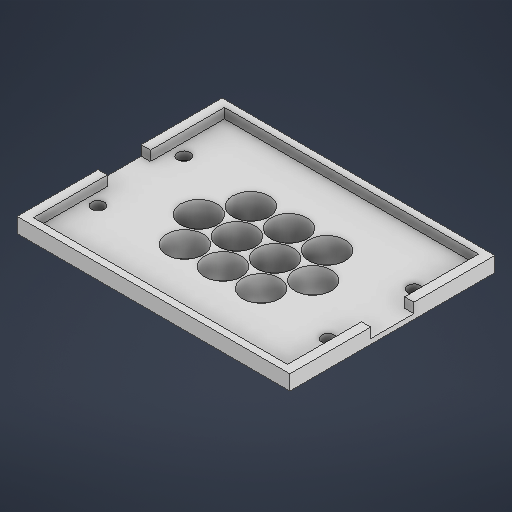
# Autodesk Inventor part: CELLCASE21700
Saved by Autodesk Inventor 2025.2 (Build 292293000, 293)
## iProperties
Created: 2025-01-16
Part Number: CELLCASE21700
Material: Generic
Document SubType Name: Modeling
Designer: cbast
Density: 1 g/cm^3
Appearance: Default
Author: cbast
## iProperties of the stored document CELLCASE21700_3DPrint.ipt
Created: 2025-01-31
Part Number: CELLCASE21700_3DPrint
Material: Generic
Document SubType Name: Modeling
Designer: cbast
Density: 1 g/cm^3
Appearance: Default
Author: cbast
Autodesk Inventor part; units mm, degrees
ref_plane "YZ Plane" through (0, 0, 0) normal (1, 0, 0) x (0, 1, 0)
ref_plane "XZ Plane" through (0, 0, 0) normal (0, 1, 0) x (-1, 0, 0)
ref_plane "XY Plane" through (0, 0, 0) normal (0, 0, 1) x (1, 0, 0)
sketch "Sketch1" plane through (0, 0, 0) normal (0, 1, 0) x (-1, 0, 0)
  circle A0 centre (0, 0) radius 11
  line L0 (11, 0.0002) -> (12, 0.0002) construction
  circle A1 centre (23, 0) radius 11
  line L1 (34, 0) -> (35, 0) construction
  circle A2 centre (46, 0) radius 11
  line L2 (57, 0) -> (58, 0) construction
  circle A3 centre (69, 0) radius 11
  line L3 (34.5, 0) -> (34.5, -17.154) construction
  line L4 (34.5, 0) -> (34.5, 17.658) construction
  line L5 (55, 12.6387) -> (55, -13.5831) construction
  line L6 (55, 12.6387) -> (55, 17.658) construction
  line L7 (55, -13.5831) -> (55, -17.154) construction
  line L8 (11.5, 0.0002) -> (11.5, -16.2579) construction
  line L9 (11.5, 0.0002) -> (11.5, 19.9186) construction
  circle A4 centre (0, 0) radius 12 construction
  circle A5 centre (23, 0) radius 12 construction
  circle A6 centre (46, 0) radius 12 construction
  circle A7 centre (69, 0) radius 12 construction
  circle A8 centre (11.5, 19.9186) radius 11
  circle A9 centre (34.5, 19.9186) radius 11
  circle A10 centre (11.5, -19.9186) radius 11
  circle A11 centre (57.5, 19.9186) radius 11
  circle A12 centre (57.5, -19.9186) radius 12 construction
  circle A13 centre (34.5, -19.9186) radius 12 construction
  circle A14 centre (11.5, 19.9186) radius 12 construction
  circle A15 centre (34.5, 19.9186) radius 12 construction
  circle A16 centre (57.5, 19.9186) radius 12 construction
  line L10 (11.5, 19.9186) -> (57.5, 19.9186) construction
  arc A17 (2.3131, -12.7926) -> (0.5, -12.9904) centre (0, 0) ccw construction
  circle A18 centre (11.5, 19.9186) radius 13 construction
  circle A19 centre (34.5, 19.9186) radius 13 construction
  circle A20 centre (57.5, 19.9186) radius 13 construction
  circle A21 centre (69, 0) radius 13 construction
  circle A22 centre (57.5, -19.9186) radius 13 construction
  circle A23 centre (34.5, -19.9186) radius 13 construction
  arc A24 (0.5, 12.9904) -> (0.5, -12.9904) centre (0, 0) ccw
  line L11 (57.5, -19.9186) -> (11.5, -19.9186) construction
  circle A25 centre (11.5, -19.9186) radius 13 construction
  arc A26 (0.5, -12.9904) -> (23, -25.9808) centre (11.5, -19.9186) ccw
  arc A27 (23, -25.9808) -> (46, -25.9808) centre (34.5, -19.9186) ccw
  arc A28 (46, -25.9808) -> (68.5, -12.9904) centre (57.5, -19.9186) ccw
  arc A29 (68.5, -12.9904) -> (68.5, 12.9904) centre (69, 0) ccw
  arc A30 (68.5, 12.9904) -> (46, 25.9808) centre (57.5, 19.9186) ccw
  arc A31 (46, 25.9808) -> (23, 25.9808) centre (34.5, 19.9186) ccw
  arc A32 (23, 25.9808) -> (0.5, 12.9904) centre (11.5, 19.9186) ccw
  circle A33 centre (11.5, -19.9186) radius 12 construction
  circle A34 centre (34.5, -19.9186) radius 11
  circle A35 centre (57.5, -19.9186) radius 11
  dimension "d0" = 22
  dimension "d6" = 22
  dimension "d1" = 1
  dimension "d2" = 22
  dimension "d3" = 1
  dimension "d4" = 22
  dimension "d5" = 1
  dimension "d7" = 24
  dimension "d8" = 24
  dimension "d9" = 24
  dimension "d10" = 24
  dimension "d11" = 22
  dimension "d12" = 22
  dimension "d16" = 22
  dimension "d17" = 22
  dimension "d19" = 24
  dimension "d21" = 24
  dimension "d22" = 24
  dimension "d23" = 24
  dimension "d25" = 26
  dimension "d27" = 26
  dimension "d28" = 26
  dimension "d29" = 26
  dimension "d30" = 26
  dimension "d31" = 26
  dimension "d32" = 26
  dimension "d33" = 26
  dimension "d67" = 24
  dimension "d71" = 24
  dimension "d72" = 22
  dimension "d73" = 22
  constraints: 37 point on circle, 34 centre point, 29 coincident, 24 end point, 12 tangent, 4 horizontal, 4 vertical, 3 midpoint, 3 point on line, 1 horizontal alignment, 6 other
  measures "d1" distance of L0.start L0.end
  measures "d2" diameter of A1
  measures "d3" distance of L1.start L1.end
  measures "d4" diameter of A2
  measures "d5" distance of L2.start L2.end
  measures "d7" diameter of A4
  measures "d8" diameter of A5
  measures "d9" diameter of A6
  measures "d10" diameter of A7
  measures "d11" diameter of A8
  measures "d12" diameter of A9
  measures "d16" diameter of A10
  measures "d17" diameter of A11
  measures "d19" diameter of A13
  measures "d21" diameter of A14
  measures "d22" diameter of A15
  measures "d23" diameter of A16
  measures "d25" diameter of A17
  measures "d27" diameter of A18
  measures "d28" diameter of A19
  measures "d29" diameter of A20
  measures "d30" diameter of A21
  measures "d31" diameter of A22
  measures "d32" diameter of A23
  measures "d33" diameter of A25
  measures "d67" diameter of A12
  measures "d71" diameter of A33
  measures "d72" diameter of A34
  measures "d73" diameter of A35
extrude "Extrusion1" add sketch "Sketch1" along normal blind 15
sketch "Sketch2" plane through (0, 15, 0) normal (0, 1, 0) x (1, 0, 0)
  circle A0 centre (-23, 0) radius 11 projected
  circle A1 centre (-46, 0) radius 11 projected
  line L0 (-35, 0) -> (-34, 0) construction
  line L1 (-111.2, 57.65) -> (42.2, 57.65)
  line L2 (42.2, 57.65) -> (42.2, -57.65)
  line L3 (42.2, -57.65) -> (-111.2, -57.65)
  line L4 (-111.2, -57.65) -> (-111.2, 57.65)
  line L5 (-111.2, 57.65) -> (42.2, -57.65) construction
  line L6 (42.2, 57.65) -> (-111.2, -57.65) construction
  arc A2 (-46, 25.9808) -> (-68.5, 12.9904) centre (-57.5, 19.9186) ccw projected
  arc A3 (-23, 25.9808) -> (-46, 25.9808) centre (-34.5, 19.9186) ccw projected
  arc A4 (-0.5, 12.9904) -> (-23, 25.9808) centre (-11.5, 19.9186) ccw projected
  arc A5 (-0.5, -12.9904) -> (-0.5, 12.9904) centre (0, 0) ccw projected
  arc A6 (-23, -25.9808) -> (-0.5, -12.9904) centre (-11.5, -19.9186) ccw projected
  arc A7 (-46, -25.9808) -> (-23, -25.9808) centre (-34.5, -19.9186) ccw projected
  arc A8 (-68.5, -12.9904) -> (-46, -25.9808) centre (-57.5, -19.9186) ccw projected
  arc A9 (-68.5, 12.9904) -> (-68.5, -12.9904) centre (-69, 0) ccw projected
  arc A10 (-69, 13) -> (-68.5, -12.9904) centre (-69, 0) ccw
  arc A11 (-46, 25.9808) -> (-68.5, 12.9904) centre (-57.5, 19.9186) ccw
  arc A12 (-23, 25.9808) -> (-46, 25.9808) centre (-34.5, 19.9186) ccw
  arc A13 (-0.5, 12.9904) -> (-23, 25.9808) centre (-11.5, 19.9186) ccw
  arc A14 (-0.5, -12.9904) -> (-0.5, 12.9904) centre (0, 0) ccw
  arc A15 (-23, -25.9808) -> (-0.5, -12.9904) centre (-11.5, -19.9186) ccw
  arc A16 (-46, -25.9808) -> (-23, -25.9808) centre (-34.5, -19.9186) ccw
  arc A17 (-68.5, -12.9904) -> (-46, -25.9808) centre (-57.5, -19.9186) ccw
  arc A18 (-68.5, 12.9904) -> (-68.5, -12.9904) centre (-69, 0) ccw
  point P0 (-34.5, 0)
  dimension "d36" = 115.3
  dimension "d37" = 153.4
  constraints: 18 point on circle, 14 end point, 9 centre point, 9 coincident, 3 midpoint, 2 horizontal, 2 horizontal alignment, 2 parallel, 1 perpendicular, 2 other
  measures "d36" distance of L3.end L1.start
  measures "d37" distance of L1.start L1.end
extrude "Extrusion2" add sketch "Sketch2" against normal blind 5 contours L1 L2 L3 L4
sketch "Sketch3" plane through (0, 15, 0) normal (0, 1, 0) x (1, 0, 0)
  line L0 (42.2, 57.65) -> (-111.2, 57.65) projected
  line L1 (42.2, -57.65) -> (42.2, 57.65) projected
  line L2 (-111.2, -57.65) -> (42.2, -57.65) projected
  line L3 (-111.2, 57.65) -> (-111.2, -57.65) projected
  line L4 (-111.2, -57.65) -> (42.2, -57.65) projected
  line L5 (42.2, -57.65) -> (42.2, 57.65) projected
  line L6 (42.2, 57.65) -> (-111.2, 57.65) projected
  line L7 (-111.2, 57.65) -> (-111.2, -57.65) projected
  circle A0 centre (-57.5, -19.9186) radius 11 projected
  circle A1 centre (-11.5, 19.9186) radius 11 projected
  circle A2 centre (-34.5, -19.9186) radius 11 projected
  circle A3 centre (-11.5, -19.9186) radius 11 projected
  circle A4 centre (-69, 0) radius 11 projected
  circle A5 centre (-46, 0) radius 11 projected
  circle A6 centre (-23, 0) radius 11 projected
  circle A7 centre (0, 0) radius 11 projected
  line L8 (-116.8026, 61.8611) -> (47.8026, 61.8611)
  line L9 (47.8026, 61.8611) -> (47.8026, -61.8611)
  line L10 (47.8026, -61.8611) -> (-116.8026, -61.8611)
  line L11 (-116.8026, -61.8611) -> (-116.8026, 61.8611)
  line L12 (-116.8026, 61.8611) -> (47.8026, -61.8611) construction
  line L13 (47.8026, 61.8611) -> (-116.8026, -61.8611) construction
  line L14 (-111.2, -57.65) -> (42.2, -57.65)
  line L15 (42.2, -57.65) -> (42.2, 57.65)
  line L16 (42.2, 57.65) -> (-111.2, 57.65)
  line L17 (-111.2, 57.65) -> (-111.2, -57.65)
  line L18 (-111.2, -57.65) -> (42.2, 57.65) construction
  line L19 (42.2, -57.65) -> (-111.2, 57.65) construction
  point P0 (-34.5, 0)
  constraints: 24 end point, 4 midpoint, 4 parallel, 3 point on line, 2 horizontal, 2 perpendicular
extrude "Extrusion3" add sketch "Sketch3" along normal blind 6 and the other way blind 3 contours L8 L9 L10 L11
sketch "Sketch4" plane through (0, 15, 0) normal (0, 1, 0) x (1, 0, 0)
  line L0 (-111.2, -57.65) -> (42.2, -57.65) projected
  line L1 (42.2, -57.65) -> (42.2, 57.65) projected
  line L2 (42.2, 57.65) -> (-111.2, 57.65) projected
  line L3 (-111.2, 57.65) -> (-111.2, -57.65) projected
  circle A0 centre (-57.5, -19.9186) radius 11 projected
  circle A1 centre (-11.5, 19.9186) radius 11 projected
  circle A2 centre (-34.5, -19.9186) radius 11 projected
  circle A3 centre (-11.5, -19.9186) radius 11 projected
  circle A4 centre (-69, 0) radius 11 projected
  circle A5 centre (-46, 0) radius 11 projected
  circle A6 centre (-23, 0) radius 11 projected
  circle A7 centre (0, 0) radius 11 projected
  line L4 (-111.2, 57.65) -> (-103.972, 57.65) construction
  line L5 (-103.972, 57.65) -> (-103.972, 25.9) construction
  line L6 (-103.972, 25.9) -> (-111.2, 25.9) construction
  line L7 (-111.2, 25.9) -> (-111.2, 57.65) construction
  line L8 (42.2, 57.65) -> (34.972, 57.65) construction
  line L9 (34.972, 57.65) -> (34.972, 25.9) construction
  line L10 (34.972, 25.9) -> (42.2, 25.9) construction
  line L11 (42.2, 25.9) -> (42.2, 57.65) construction
  line L12 (-111.2, -57.65) -> (-103.972, -57.65) construction
  line L13 (-103.972, -57.65) -> (-103.972, -25.9) construction
  line L14 (-103.972, -25.9) -> (-111.2, -25.9) construction
  line L15 (-111.2, -25.9) -> (-111.2, -57.65) construction
  line L16 (42.2, -25.9) -> (34.972, -25.9) construction
  line L17 (34.972, -25.9) -> (34.972, -57.65) construction
  line L18 (34.972, -57.65) -> (42.2, -57.65) construction
  line L19 (42.2, -57.65) -> (42.2, -25.9) construction
  circle A8 centre (-103.972, 25.9) radius 3.865
  circle A9 centre (34.972, 25.9) radius 3.865
  circle A10 centre (34.972, -25.9) radius 3.865
  circle A11 centre (-103.972, -25.9) radius 3.865
  dimension "d56" = 7.73
  dimension "d57" = 7.73
  dimension "d58" = 7.73
  dimension "d59" = 7.73
  dimension "d62" = 7.228
  dimension "d63" = 31.75
  dimension "d64" = 7.228
  dimension "d65" = 7.228
  dimension "d66" = 31.75
  constraints: 32 end point, 8 parallel, 5 point on line, 4 centre point, 4 coincident, 4 horizontal, 4 perpendicular
  measures "d56" diameter of A9
  measures "d57" diameter of A8
  measures "d58" diameter of A11
  measures "d59" diameter of A10
  measures "d62" distance of L5.end L6.end
  measures "d63" distance of L4.end L5.end
  measures "d64" distance of L9.end L10.end
  measures "d65" distance of L16.start L16.end
  measures "d66" distance of L16.end L17.end
extrude "Extrusion4" cut sketch "Sketch4" against normal through all contours A8 | A9 | A10 | A11
sketch "Sketch5" plane through (-116.8026, 12, 61.8611) normal (-1, 0, 0) x (0, 0, 1)
  line L0 (-74.8611, -12) -> (-74.8611, -2) projected
  line L1 (-48.8611, -12) -> (-48.8611, -2) projected
  line L2 (-119.5111, 3) -> (-4.2111, 3) projected
  line L3 (-123.7222, 9) -> (0, 9) projected
  line L4 (-74.8611, 3) -> (-48.8611, 3)
  line L5 (-48.8611, 3) -> (-48.8611, 9)
  line L6 (-48.8611, 9) -> (-74.8611, 9)
  line L7 (-74.8611, 9) -> (-74.8611, 3)
  point P0 (-61.8611, -12)
  constraints: 8 end point, 2 parallel, 2 point on line, 1 horizontal, 1 perpendicular
extrude "Extrusion5" cut sketch "Sketch5" against normal through all
body "Solid1"
